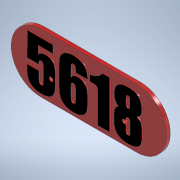
# Autodesk Inventor part: 5618 v3
Saved by Autodesk Inventor 2022 (Build 260153000, 153)
## iProperties
Created: 2021-11-18
Part Number: 5618 v3
Material: Generic
Document SubType Name: Modeling
Designer: TakeHomePC
Density: 1 g/cm^3
Appearance: Default
Author: TakeHomePC
Autodesk Inventor part; units mm, degrees
ref_plane "YZ Plane" through (0, 0, 0) normal (1, 0, 0) x (0, 1, 0)
ref_plane "XZ Plane" through (0, 0, 0) normal (0, 1, 0) x (-1, 0, 0)
ref_plane "XY Plane" through (0, 0, 0) normal (0, 0, 1) x (1, 0, 0)
sketch "Sketch2" plane through (0, 0, 0) normal (0, 0, 1) x (1, 0, 0)
  line L0 (20.8189, 49.0215) -> (188.5216, 49.0215) construction
  line L1 (188.5216, 49.0215) -> (188.5216, -14.4785) construction
  line L2 (188.5216, -14.4785) -> (20.8189, -14.4785) construction
  line L3 (20.8189, -14.4785) -> (20.8189, 49.0215) construction
  line L4 (39.7523, -23.1809) -> (169.7523, -23.1809)
  line L5 (169.7523, 56.3191) -> (39.7523, 56.3191)
  arc A0 (39.7523, 56.3191) -> (39.7523, -23.1809) centre (39.7523, 16.5691) ccw
  arc A1 (169.7523, -23.1809) -> (169.7523, 56.3191) centre (169.7523, 16.5691) ccw
  line L6 (39.7523, 16.5691) -> (169.7523, 16.5691) construction
  line L7 (13.9504, -10.894) -> (193.9504, -10.894)
  line L8 (193.9504, -10.894) -> (193.9504, 37.106)
  line L9 (193.9504, 37.106) -> (13.9504, 37.106)
  line L10 (13.9504, 37.106) -> (13.9504, -10.894)
  line L11 (13.9504, -10.894) -> (193.9504, 37.106) construction
  line L12 (193.9504, -10.894) -> (13.9504, 37.106) construction
  circle A2 centre (55.9046, 6.35) radius 2.85
  circle A3 centre (154.5639, 6.35) radius 2.85
  circle A4 centre (55.9046, 43.9691) radius 4
  circle A5 centre (55.9046, -17.1809) radius 4
  circle A6 centre (154.5639, -17.1809) radius 4
  circle A7 centre (154.5639, 43.9691) radius 4
  line L13 (154.5639, 43.9691) -> (154.5639, -17.1809) construction
  line L14 (55.9046, -17.1809) -> (55.9046, 43.9691) construction
  line L15 (58.2394, 47.7295) -> (58.2394, 37.5848)
  line L16 (58.2394, 37.5848) -> (38.5721, 37.5848)
  line L17 (38.5721, 37.5848) -> (38.5721, 26.7702)
  spline S0 degree 2 poles (38.5721, 26.7702) (42.2568, 31.1247) (48.0948, 31.1247) knots 0 0 0 1 1 1
  spline S1 degree 2 poles (48.0948, 31.1247) (54.6505, 31.1247) (61.3498, 23.8033) (61.3498, 13.3715) knots 0 0 0 1 2 2 2
  line L18 (61.3498, 13.3715) -> (61.3498, 4.3275)
  spline S2 degree 2 poles (61.3498, 4.3275) (61.3498, -2.4197) (60.0578, -8.7362) (55.799, -14.0957) (48.2383, -16.9668) (42.7831, -16.9668) knots 0 0 0 1 2 3 4 4 4
  spline S3 degree 2 poles (42.7831, -16.9668) (36.6581, -16.9668) (27.3269, -12.708) (23.403, -4.2381) (23.403, 4.6146) knots 0 0 0 1 2 3 3 3
  line L19 (23.403, 4.6146) -> (23.403, 8.0599)
  line L20 (23.403, 8.0599) -> (39.2421, 8.0599)
  line L21 (39.2421, 8.0599) -> (39.2421, 4.0882)
  spline S4 degree 2 poles (39.2421, 4.0882) (39.2421, -2.0369) (40.1034, -7.205) (42.6874, -7.205) knots 0 0 0 1 2 2 2
  spline S5 degree 2 poles (42.6874, -7.205) (43.8359, -7.205) (45.3193, -5.7215) (45.415, -3.9988) (45.5107, 2.6526) knots 0 0 0 1 2 3 3 3
  line L22 (45.5107, 2.6526) -> (45.5107, 15.1899)
  spline S6 degree 2 poles (45.5107, 15.1899) (45.5107, 18.7788) (44.0273, 21.3629) (42.2568, 21.3629) knots 0 0 0 1 2 2 2
  spline S7 degree 2 poles (42.2568, 21.3629) (41.1562, 21.3629) (39.6727, 20.023) (39.2421, 18.4917) (39.2421, 15.7163) knots 0 0 0 1 2 3 3 3
  line L23 (39.2421, 15.7163) -> (23.5465, 15.7163)
  line L24 (23.5465, 15.7163) -> (24.2165, 47.7295)
  line L25 (24.2165, 47.7295) -> (58.2394, 47.7295)
  line L26 (104.7997, 30.8855) -> (88.9606, 30.8855)
  spline S8 degree 2 poles (88.9606, 30.8855) (88.9606, 35.3357) (88.7692, 37.6327) (87.0944, 39.2118) (85.611, 39.2118) knots 0 0 0 1 2 3 3 3
  spline S9 degree 2 poles (85.611, 39.2118) (84.4146, 39.2118) (82.8355, 37.7284) (82.5963, 35.3836) (82.5963, 31.7947) knots 0 0 0 1 2 3 3 3
  line L27 (82.5963, 31.7947) -> (82.5963, 21.65)
  spline S10 degree 2 poles (82.5963, 21.65) (83.7926, 24.234) (88.5299, 26.7702) (91.9753, 26.7702) knots 0 0 0 1 2 2 2
  spline S11 degree 2 poles (91.9753, 26.7702) (96.3299, 26.7702) (102.9813, 22.0807) (104.7997, 15.477) (104.7997, 9.8783) knots 0 0 0 1 2 3 3 3
  line L28 (104.7997, 9.8783) -> (104.7997, 4.806)
  spline S12 degree 2 poles (104.7997, 4.806) (104.7997, -1.8455) (103.7948, -8.3534) (99.3446, -13.9043) (91.6403, -16.9668) (86.4723, -16.9668) knots 0 0 0 1 2 3 4 4 4
  spline S13 degree 2 poles (86.4723, -16.9668) (80.1079, -16.9668) (71.9252, -13.4258) (67.5228, -6.8221) (66.7571, 0.4993) (66.7571, 11.0268) knots 0 0 0 1 2 3 4 4 4
  line L29 (66.7571, 11.0268) -> (66.7571, 19.7837)
  spline S14 degree 2 poles (66.7571, 19.7837) (66.7571, 31.1247) (67.4271, 38.7811) (72.2123, 45.624) (80.4908, 49.0215) (85.8981, 49.0215) knots 0 0 0 1 2 3 4 4 4
  spline S15 degree 2 poles (85.8981, 49.0215) (92.5495, 49.0215) (101.1151, 44.7148) (104.7997, 36.867) (104.7997, 30.8855) knots 0 0 0 1 2 3 3 3
  spline S16 degree 2 poles (88.9606, 11.0746) (88.9606, 14.4721) (87.4772, 16.9605) (85.8024, 16.9605) knots 0 0 0 1 2 2 2
  spline S17 degree 2 poles (85.8024, 16.9605) (84.1275, 16.9605) (82.5963, 14.5678) (82.5963, 11.0746) knots 0 0 0 1 2 2 2
  line L30 (82.5963, 11.0746) -> (82.5963, -0.4099)
  spline S18 degree 2 poles (82.5963, -0.4099) (82.5963, -4.6209) (84.0318, -7.205) (85.7545, -7.205) knots 0 0 0 1 2 2 2
  spline S19 degree 2 poles (85.7545, -7.205) (86.7594, -7.205) (88.9606, -5.1952) (88.9606, -0.7927) knots 0 0 0 1 2 2 2
  line L31 (88.9606, -0.7927) -> (88.9606, 11.0746)
  line L32 (134.6596, 47.7295) -> (134.6596, -15.7705)
  line L33 (134.6596, -15.7705) -> (118.8204, -15.7705)
  line L34 (118.8204, -15.7705) -> (118.8204, 18.3003)
  spline S20 degree 2 poles (118.8204, 18.3003) (118.8204, 25.6696) (118.1027, 28.6364) (114.9444, 30.1677) (109.4892, 30.1677) knots 0 0 0 1 2 3 3 3
  line L35 (109.4892, 30.1677) -> (107.9101, 30.1677)
  line L36 (107.9101, 30.1677) -> (107.9101, 37.5848)
  spline S21 degree 2 poles (107.9101, 37.5848) (119.3947, 40.0253) (125.3762, 47.7295) knots 0 0 0 1 1 1
  line L37 (125.3762, 47.7295) -> (134.6596, 47.7295)
  spline S22 degree 2 poles (171.0752, 20.3101) (174.5684, 18.8746) (178.3487, 13.2758) (178.3487, 2.7005) knots 0 0 0 1 2 2 2
  spline S23 degree 2 poles (178.3487, 2.7005) (178.3487, -5.0037) (175.3819, -12.2773) (166.7206, -16.9668) (159.4949, -16.9668) knots 0 0 0 1 2 3 3 3
  spline S24 degree 2 poles (159.4949, -16.9668) (152.4128, -16.9668) (144.1822, -12.4687) (140.5932, -5.0995) (140.5932, 3.4661) knots 0 0 0 1 2 3 3 3
  spline S25 degree 2 poles (140.5932, 3.4661) (140.5932, 9.2562) (142.3638, 17.7261) (147.0533, 20.3101) knots 0 0 0 1 2 2 2
  spline S26 degree 2 poles (147.0533, 20.3101) (144.0865, 21.6978) (141.1675, 27.8708) (141.1675, 32.6082) knots 0 0 0 1 2 2 2
  spline S27 degree 2 poles (141.1675, 32.6082) (141.1675, 40.7909) (150.2594, 48.9736) (159.3035, 48.9736) knots 0 0 0 1 2 2 2
  spline S28 degree 2 poles (159.3035, 48.9736) (169.7831, 48.9736) (177.7745, 40.2645) (177.7745, 32.1775) knots 0 0 0 1 2 2 2
  spline S29 degree 2 poles (177.7745, 32.1775) (177.7745, 27.0573) (175.1426, 22.5113) (171.0752, 20.3101) knots 0 0 0 1 2 2 2
  spline S30 degree 2 poles (162.5096, 7.5336) (162.5096, 11.1703) (161.0262, 13.5629) (159.3992, 13.5629) knots 0 0 0 1 2 2 2
  spline S31 degree 2 poles (159.3992, 13.5629) (157.8201, 13.5629) (156.4324, 11.266) (156.4324, 7.5336) knots 0 0 0 1 2 2 2
  line L38 (156.4324, 7.5336) -> (156.4324, -0.7449)
  spline S32 degree 2 poles (156.4324, -0.7449) (156.4324, -4.8602) (157.9636, -7.205) (159.6385, -7.205) knots 0 0 0 1 2 2 2
  spline S33 degree 2 poles (159.6385, -7.205) (161.3133, -7.205) (162.5096, -4.8123) (162.5096, -0.6013) knots 0 0 0 1 2 2 2
  line L39 (162.5096, -0.6013) -> (162.5096, 7.5336)
  spline S34 degree 2 poles (162.1746, 33.9002) (162.1746, 37.1541) (161.0262, 39.2118) (159.447, 39.2118) knots 0 0 0 1 2 2 2
  spline S35 degree 2 poles (159.447, 39.2118) (157.8679, 39.2118) (156.7673, 36.9627) (156.7673, 33.9002) knots 0 0 0 1 2 2 2
  line L40 (156.7673, 33.9002) -> (156.7673, 29.1149)
  spline S36 degree 2 poles (156.7673, 29.1149) (156.7673, 26.2438) (158.0115, 24.0426) (159.4949, 24.0426) knots 0 0 0 1 2 2 2
  spline S37 degree 2 poles (159.4949, 24.0426) (161.074, 24.0426) (162.1746, 26.196) (162.1746, 29.5935) knots 0 0 0 1 2 2 2
  line L41 (162.1746, 29.5935) -> (162.1746, 33.9002)
  point P0 (0, 0)
  point P1 (103.9504, 13.106)
  dimension "d33" = 79.5
  dimension "d35" = 130
  dimension "d40" = 63.5
  dimension "d41" = 48
  dimension "d42" = 180
  dimension "d43" = 5.7
  dimension "d44" = 5.7
  dimension "d47" = 8
  constraints: 22 end point, 8 centre point, 4 point on circle, 4 tangent, 3 equal radius, 3 parallel, 3 perpendicular, 2 midpoint, 2 point on line, 1 horizontal, 6 other
  measures "d33" distance between parallel lines of L4 L5
  measures "d35" distance of L6.end L6.start
  measures "d40" distance between parallel lines of L2 L0
  measures "d41" distance of L8.end L7.end
  measures "d42" distance between parallel lines of L8 L10
  measures "d43" diameter of A2
  measures "d44" diameter of A3
  measures "d47" diameter of A4
extrude "Extrusion4" add sketch "Sketch2" along normal blind 2 contours S3 L19 L20 L21 S4 S5 L22 S6 S7 L23 L24 L9 L17 S0 S1 L18 S2 L7 | L7 S2 A5 S3 | L24 L25 A4 L15 L16 L17 L9 | S13 L29 S14 L9 S9 L27 S10 S11 L28 S12 L7 | L7 S12 S13 | S2 A5 | S14 S15 L9 S8 S9 | L25 A4 L15 | L34 S20 L35 L36 L9 L32 L7 | L7 L32 L33 L34 | L25 L15 A4 | L9 S15 L26 S8 | S24 S25 S26 S27 L9 S35 L40 S36 S37 L41 S34 S28 S29 S22 S23 L7 | L7 S23 S24 A6 | L9 L36 S21 L37 L32 | A6 S24 | S27 S28 L9 S34 S35 | A2 | S31 L38 A3 | A7 picked at (53.1786, -14.8183) picked at (157.1014, -16.5184) picked at (153.5127, 5.8753)
extrude "Extrusion7" add sketch "Sketch2" against normal blind 5 from surface at 0 contours A0 L5 A1 L4 | L10 L9 L24 L23 S7 S6 L22 S5 S4 L21 L20 L19 S3 L7 | S3 L19 L20 L21 S4 S5 L22 S6 S7 L23 L24 L9 L17 S0 S1 L18 S2 L7 | L7 S2 A5 S3 | S2 L18 S1 S0 L17 L9 S14 L29 S13 L7 | L24 L25 A4 L15 L16 L17 L9 | S13 L29 S14 L9 S9 L27 S10 S11 L28 S12 L7 | L7 S12 S13 | S2 A5 | A5 S2 | S12 L28 S11 S10 L27 S9 L9 S8 L26 S15 L36 L35 S20 L34 L7 | S14 S15 L9 S8 S9 | L25 A4 L15 | A4 L25 | L34 S20 L35 L36 L9 L32 L7 | L7 L32 L33 L34 | S9 S8 L9 | L25 L15 A4 | L15 A4 | L32 L9 S27 S26 S25 S24 L7 | L9 S15 L26 S8 | S24 S25 S26 S27 L9 S35 L40 S36 S37 L41 S34 S28 S29 S22 S23 L7 | L7 S23 S24 A6 | L9 L36 S21 L37 L32 | S23 S22 S29 S28 L9 L8 L7 | S24 A6 | A6 S24 | S27 S28 L9 S34 S35 | S35 S34 L9 | L9 S34 L41 S37 S36 L40 S35 | A3 S31 S30 L39 S33 S32 L38 | A7 | L31 S19 S18 L30 S17 S16
extrude "Extrusion9" cut sketch "Sketch2" along normal through all contours A2 | A3 L38 S31 | S31 L38 A3
extrude "Extrusion10" cut sketch "Sketch2" along normal blind 3.5 from surface at -5 contours S2 A5 | A5 S2 | L25 A4 L15 | A4 L25 | L15 A4 | S24 A6 | A6 S24 | A7 picked at (56.7959, 45.3465)
chamfer "Chamfer1" distance 3 angle 45 4 edges at (51.9046, 43.9691, -5) (51.9046, -17.1809, -5) (150.5639, 43.9691, -5) (150.5639, -17.1809, -5)
body "Solid3"
